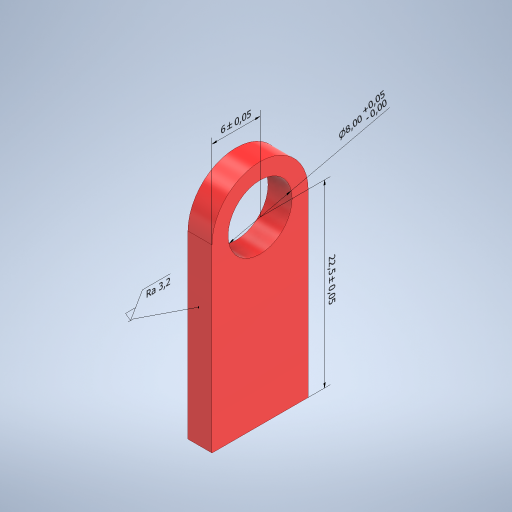
# Autodesk Inventor part: rapoukMiddleLeg1v3
Saved by Autodesk Inventor 2024 (Build 280153000, 153)
## iProperties
Created: 2023-05-29
Part Number: rapoukMiddleLeg1v3
Material: EN AW-6060 T6
Document SubType Name: Modeling
Designer: Roman
Density: 2.7 g/cm^3
Appearance: Light Red
Mass: 2.13183 g
Surface Area: 8.76112 cm^2
Volume: 0.789566 cm^3
Description: Nehybná část nohy
Polotovar: KR...
Author: Roman
## iProperties of the stored document middleLegv2-1_3DPrint.ipt
Created: 2023-06-18
Part Number: middleLegv2-1_3DPrint
Material: Generic
Document SubType Name: Modeling
Designer: Roman
Density: 1 g/cm^3
Appearance: Default
Author: Roman
Autodesk Inventor part; units mm, degrees
ref_plane "YZ Plane" through (0, 0, 0) normal (1, 0, 0) x (0, 1, 0)
ref_plane "XZ Plane" through (0, 0, 0) normal (0, 1, 0) x (-1, 0, 0)
ref_plane "XY Plane" through (0, 0, 0) normal (0, 0, 1) x (1, 0, 0)
sketch "Sketch1" plane through (0, 0, 0) normal (0, 1, 0) x (-1, 0, 0)
  line L0 (-1.5, 6) -> (1.5, 6)
  line L1 (1.5, 6) -> (1.5, -6)
  line L2 (1.5, -6) -> (-1.5, -6)
  line L3 (-1.5, -6) -> (-1.5, 6)
  line L4 (-1.5, 6) -> (1.5, -6) construction
  line L5 (1.5, 6) -> (-1.5, -6) construction
  point P0 (0, 0)
  dimension "d0" = 3
  dimension "d1" = 12
  constraints: 12 end point, 2 midpoint, 2 parallel, 1 horizontal, 1 perpendicular
  measures "d0" distance of L1.end L2.end
  measures "d1" distance of L0.end L1.end
extrude "Extrusion1" add sketch "Sketch1" along normal blind 28.5
fillet "Fillet1" radius 6 2 edges at (0, 28.5, 6) (0, 28.5, -6)
sketch "Sketch4" plane through (1.5, 0, 6) normal (1, 0, 0) x (0, 0, -1)
  arc A0 (12, 22.5) -> (0, 22.5) centre (6, 22.5) ccw projected
  circle A1 centre (6, 22.5) radius 4
  point P0 (6, 0)
  dimension "d14" = 8
  constraints: 1 centre point, 1 coincident
  measures "d14" diameter of A1
extrude "Extrusion4" cut sketch "Sketch4" against normal through all
body "Solid1"
